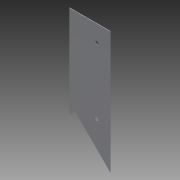
# Autodesk Inventor part: Plate_InnerSide_Alu25
Saved by Autodesk Inventor 2013 (Build 170138000, 138)
## iProperties
Created: 2015-07-02
Part Number: Plate_InnerSide_Alu25
Material: Aluminum 6061
Document SubType Name: Modeling
Designer: Kyle
Density: 2.71 g/cm^3
Mass: 4.1528 g
Surface Area: 69.1305 cm^2
Volume: 1.5324 cm^3
Author: Kyle
Autodesk Inventor part; units mm, degrees
ref_plane "YZ Plane" through (0, 0, 0) normal (1, 0, 0) x (0, 1, 0)
ref_plane "XZ Plane" through (0, 0, 0) normal (0, 1, 0) x (-1, 0, 0)
ref_plane "XY Plane" through (0, 0, 0) normal (0, 0, 1) x (1, 0, 0)
sketch "Sketch1" plane through (0, 0, 0) normal (0, 0, 1) x (1, 0, 0)
  line L0 (0, 0) -> (38.1, 0)
  line L1 (38.1, 0) -> (38.1, -85.725)
  line L2 (38.1, -85.725) -> (0, -85.725)
  line L3 (0, -85.725) -> (0, 0)
  line L4 (38.1, -85.725) -> (38.1, -123.825)
  line L5 (38.1, -123.825) -> (0, -85.725)
  dimension "d0" = 38.1
  dimension "d1" = 85.725
  dimension "d4" = 38.1
  constraints: 12 end point, 3 parallel, 1 horizontal, 1 perpendicular
  measures "d0" distance of L0.start L0.end
  measures "d1" distance of L2.end L0.start
  measures "d4" distance of L1.end L4.end
extrude "Extrusion1" add sketch "Sketch1" along normal blind 0.4039 contours L0 L1 L2 L3
extrude "Extrusion2" add sketch "Sketch1" along normal blind 0.4039 contours L2 L4 L5
sketch "Sketch2" plane through (0, 0, 0.4039) normal (0, 0, 1) x (1, 0, 0)
  line L0 (0, -85.725) -> (38.1, -123.825) projected
  line L1 (38.1, -123.825) -> (38.1, 0) projected
  line L2 (38.1, -113.0487) -> (5.3882, -80.3368)
  line L3 (0, -85.725) -> (5.3882, -80.3368)
  line L4 (38.1, -113.0487) -> (38.1, -123.825)
  line L5 (38.1, -123.825) -> (0, -85.725)
  line L6 (0, -85.725) -> (5.3882, -80.3368)
  line L7 (5.3882, -80.3368) -> (38.1, -113.0487)
  line L8 (38.1, -113.0487) -> (38.1, -123.825)
  line L9 (38.1, -123.825) -> (0, -85.725)
  dimension "d7" = 7.62
  constraints: 16 end point, 5 collinear, 2 perpendicular, 1 parallel, 1 point on line
  measures "d7" distance between parallel lines of L0 L2
extrude "Extrusion3" cut sketch "Sketch2" against normal blind 25.4
sketch "Sketch3" plane through (0, 0, 0) normal (0, 0, -1) x (-1, 0, 0)
  circle A0 centre (-25.4, -15.24) radius 1.4986
  circle A1 centre (-25.4, -76.2) radius 1.4986
  line L0 (0, 0) -> (-38.1, 0) projected
  line L1 (-38.1, 0) -> (-38.1, -113.0487) projected
  dimension "d19" = 2.9972
  dimension "d20" = 15.24
  dimension "d21" = 12.7
  dimension "d22" = 12.7
  constraints: 2 centre point
  measures "d19" diameter of A0
  measures "d20" distance from line of L0 A0.centre
  measures "d21" distance from line of L1 A0.centre
  measures "d22" distance from line of L1 A1.centre
extrude "Extrusion4" cut sketch "Sketch3" against normal blind 25.4
body "Solid1"
